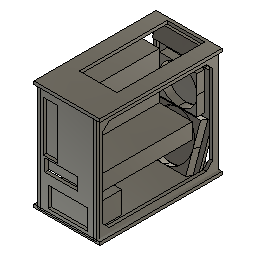
case (Autodesk Fusion 360 design; units mm, degrees)
Autodesk Fusion 360 part; units mm, degrees
sketch "Skizze1" plane through (0, 0, 0) normal (0, 1, 0) x (1, 0, 0)
  line L0 (-1.5, -33) -> (-1.5, -13)
  line L1 (-1.5, -13) -> (15.5, -13)
  line L2 (15.5, -13) -> (15.5, -18)
  line L3 (15.5, -18) -> (5, -18)
  line L4 (5, -18) -> (5, -33)
  line L5 (5, -33) -> (-1.5, -33)
  dimension "d1" = 20
  dimension "d2" = 17
  dimension "d3" = 5
  dimension "d4" = 10.5
  constraint vertical L0
  constraint perpendicular L0 L1
  constraint perpendicular L1 L2
  constraint perpendicular L0 L3
  constraint perpendicular L3 L4
  constraint perpendicular L0 L5
  measures "d1" distance of L0.start L0.end
  measures "d2" distance of L0.end L1.end
  measures "d3" distance of L1.end L2.end
  measures "d4" distance of L2.end L3.end
sketch "Skizze3" plane through (0, 0, 0) normal (1, 0, 0) x (0, 1, 0)
  line L0 (25, 35, -2) -> (-14, 35, -2)
  line L1 (-14, 35, -2) -> (-14, 1.5, -2)
  line L2 (-14, 1.5, -2) -> (25, 1.5, -2)
  line L3 (25, 1.5, -2) -> (25, 35, -2)
  line L4 (23, 31, -2) -> (21, 33, -2)
  line L5 (21, 33, -2) -> (-10, 33, -2)
  line L6 (-10, 33, -2) -> (-12, 31, -2)
  line L7 (-12, 31, -2) -> (-12, 5.5, -2)
  line L8 (-12, 5.5, -2) -> (-10, 3.5, -2)
  line L9 (-10, 3.5, -2) -> (21, 3.5, -2)
  line L10 (21, 3.5, -2) -> (23, 5.5, -2)
  line L11 (23, 5.5, -2) -> (23, 31, -2)
  line L12 (21, 33, -2) -> (23, 33, -2) construction
  line L13 (23, 31, -2) -> (23, 33, -2) construction
  line L14 (-12, 31, -2) -> (-12, 33, -2) construction
  line L15 (-12, 33, -2) -> (-10, 33, -2) construction
  line L16 (-12, 5.5, -2) -> (-12, 3.5, -2) construction
  line L17 (-12, 3.5, -2) -> (-10, 3.5, -2) construction
  line L18 (21, 3.5, -2) -> (23, 3.5, -2) construction
  line L19 (23, 3.5, -2) -> (23, 5.5, -2) construction
  dimension "d32" = 39
  dimension "height" = 33.5
  dimension "d34" = 29.5
  dimension "d35" = 35
  dimension "d36" = 2
  dimension "d37" = 2
  dimension "d38" = 2
  dimension "d39" = 2
  dimension "d40" = 2
  dimension "d41" = 2
  dimension "d42" = 2
  dimension "d43" = 2
sketch "Skizze4" plane through (0, 0, 0) normal (0, 0, 1) x (1, 0, 0)
  line L0 (-3, 25, 2) -> (18, 25, 2)
  line L1 (18, 25, 2) -> (18, -14, 2)
  line L2 (18, -14, 2) -> (-3, -14, 2)
  line L3 (-3, -14, 2) -> (-3, 25, 2)
  line L4 (13.5, -4, 2) -> (1.5, -4, 2)
  line L5 (1.5, -4, 2) -> (1.5, 24, 2)
  line L6 (1.5, 24, 2) -> (13.5, 24, 2)
  line L7 (13.5, 24, 2) -> (13.5, -4, 2)
  dimension "length" = 39
  dimension "width" = 21
sketch "Skizze5" plane through (0, 0, 0) normal (0, 1, 0) x (1, 0, 0)
  line L0 (-2, -35, -5) -> (17, -35, -5)
  line L1 (17, -35, -5) -> (17, -1.5, -5)
  line L2 (17, -1.5, -5) -> (-2, -1.5, -5)
  line L3 (-2, -1.5, -5) -> (-2, -35, -5)
  line L4 (14, -3, -5) -> (1.5, -3, -5)
  line L5 (1.5, -3, -5) -> (1.5, -9.5, -5)
  line L6 (1.5, -9.5, -5) -> (14, -9.5, -5)
  line L7 (14, -9.5, -5) -> (14, -3, -5)
  line L8 (0, -33, -5) -> (4.5, -33, -5)
  line L9 (4.5, -33, -5) -> (4.5, -17, -5)
  line L10 (4.5, -17, -5) -> (0, -17, -5)
  line L11 (0, -17, -5) -> (0, -33, -5)
  line L12 (0.5, -16.5, -5) -> (11, -16.5, -5)
  line L13 (11, -16.5, -5) -> (11, -12.5, -5)
  line L14 (11, -12.5, -5) -> (0.5, -12.5, -5)
  line L15 (0.5, -12.5, -5) -> (0.5, -16.5, -5)
  line L16 (14, -2, -5) -> (1, -2, -5)
  line L17 (1, -2, -5) -> (1, -9, -5)
  line L18 (1, -9, -5) -> (14, -9, -5)
  line L19 (14, -9, -5) -> (14, -2, -5)
  line L20 (18, -2) -> (-3, -2)
  dimension "d9" = 12.5
  dimension "d10" = 6.5
  dimension "d11" = 16
  dimension "d12" = 4.5
  dimension "d13" = 10.5
  dimension "d14" = 4
  dimension "d70" = 21
  dimension "d71" = 33.5
  measures "d70" distance of L20.start L20.end
sketch "Skizze6" plane through (0, 0, 0) normal (1, 0, 0) x (0, 1, 0)
  line L0 (25, 15.1374, -1) -> (20.2117, 1.9817, -1)
  line L1 (24, 15.1374, -1) -> (19.2117, 1.9817, -1)
  line L2 (24, 15.1374, -1) -> (24, 29.1374, -1)
  line L3 (19.2117, 1.9817, -1) -> (20.2117, 1.9817, -1)
  line L4 (25, 29.1374, -1) -> (25, 15.1374, -1)
  line L5 (22.851, 31.0958, -1) -> (24.3572, 35.234, -1)
  line L6 (24.2721, 35, -1) -> (23.1436, 35, -1)
  line L7 (23.1436, 35, -1) -> (21.7147, 31.074, -1)
  line L8 (24, 29.1323, -1) -> (21.7147, 31.074, -1)
  line L9 (25, 29.1374, -1) -> (22.851, 31.0958, -1)
  dimension "fansize" = 14
  dimension "d19" = 14
  dimension "d62" = 14
  dimension "d63" = 14
extrude "Extrusion2" add sketch "Skizze1" along normal blind 31 makes body 1
move_body "Verschieben3" bodies 1 to x (1, 0, 0) y (0, 1, 0) z (0, 0, 1) at (0, -4, 0)
extrude "Extrusion6" add sketch "Skizze5" along normal blind 1 separate body contours L0 L1 L2 L3 | L4 L5 L16 L17 L18 L19 in plane through (0, -5, 0) normal (0, 1, 0) makes body 2
move_body "Verschieben4" bodies 2 1 to x (1, 0, 0) y (0, 1, 0) z (0, 0, 1) at (0, -9, 0)
extrude "Extrusion3" add sketch "Skizze4" along normal blind 1 separate body contours L0 L1 L2 L3 in plane through (0, 0, 2) normal (0, 0, 1) makes body 3
move_body "Verschieben1" bodies 3 to x (1, 0, 0) y (0, 1, 0) z (0, 0, 1) at (0, 0, 33)
extrude "Extrusion4" add sketch "Skizze4" against normal blind 1 separate body contours L0 L1 L2 L3 | L4 L5 L6 L7 in plane through (0, 0, 2) normal (0, 0, 1) makes body 4
extrude "Extrusion5" add sketch "Skizze3" along normal blind 1 separate body contours L0 L1 L2 L3 in plane through (-2, 0, 0) normal (1, 0, 0) makes body 5
copy_body "Körper kopieren/einfügen1" bodies 5 makes body 6
move_body "Verschieben2" bodies 6 to x (1, 0, 0) y (0, 1, 0) z (0, 0, 1) at (18, 0, 0)
extrude "Extrusion7" add sketch "Skizze6" along normal blind 17 separate body contours L0 L1 L2 L3 L4 L5 L6 L7 L8 L9 in plane through (-1, 0, 0) normal (1, 0, 0) makes body 7
sketch "Skizze8" plane through (0, 16.3275, -5.9427) normal (0, -0.939693, 0.34202) x (1, 0, 0)
  line L0 (-1, 22.433) -> (-1, 8.433)
  line L1 (-1, 8.433) -> (16, 8.433)
  line L2 (16, 8.433) -> (16, 22.433)
  line L3 (16, 22.433) -> (-1, 22.433)
  circle A0 centre (7.5, 15.5) radius 7
  line L4 (0.5, 22.5) -> (14.5, 22.5)
  line L5 (14.5, 22.5) -> (14.5, 8.5)
  line L6 (14.5, 8.5) -> (0.5, 8.5)
  line L7 (0.5, 8.5) -> (0.5, 22.5)
  dimension "d57" = 14
  constraint horizontal L4
  constraint vertical L5
  constraint horizontal L6
  constraint vertical L7
  measures "d57" diameter of A0
extrude "Extrusion11" add sketch "Skizze8" along normal blind 2.5 separate body contours L3 A0 L4 L7 | L3 A0 L7 | A0 L6 L7 | L3 A0 L4 L5 | L3 A0 L5 | A0 L5 L6 makes body 8
extrude "Extrusion12" add sketch "Skizze5" along normal blind 10 separate body contours L4 L5 L7 L18 L19 | L4 L5 L16 L17 L18 L19 in plane through (0, -5, 0) normal (0, 1, 0) makes body 9
move_body "Verschieben5" bodies 9 to x (1, 0, 0) y (0, 1, 0) z (0, 0, 1) at (0, -8, 0)
sketch "Skizze9" plane through (0, 24, 0) normal (0, -1, 0) x (1, 0, 0)
  line L0 (-1, 29.1323) -> (-1, 15.1374)
  line L1 (-1, 15.1374) -> (16, 15.1374)
  line L2 (16, 15.1374) -> (16, 29.1323)
  line L3 (1.5, 28.5) -> (13.5, 28.5)
  line L4 (13.5, 28.5) -> (13.5, 16.5)
  line L5 (13.5, 16.5) -> (1.5, 16.5)
  line L6 (1.5, 16.5) -> (1.5, 28.5)
  circle A0 centre (7.5, 22.5) radius 6
  line L7 (16, 29.1323) -> (-1, 29.1323)
  dimension "d65" = 12
  dimension "d66" = 12
  dimension "d67" = 12
  constraint horizontal L3
  constraint vertical L4
  constraint horizontal L5
  constraint vertical L6
  measures "d65" distance of L3.start L3.end
  measures "d66" distance of L3.start L5.end
  measures "d67" diameter of A0
extrude "Extrusion13" add sketch "Skizze9" along normal blind 2.5 separate body contours L3 L6 A0 | L3 L4 A0 | L5 L6 A0 | L4 L5 A0 makes body 10
equation "d19 = fansize"
equation "d22 = thickness"
equation "d24 = -thickness"
equation "d26 = thickness"
equation "thickness = 1 mm"
equation "d32 = length"
equation "d34 = height - 4 mm"
equation "d35 = length - 4 mm"
equation "d44 = width - 4 mm"
equation "fan_thickness = 2.50 mm"
equation "d71 = height"
named bodies: "board", "top", "bottom", "side1", "side2", "back", "front", "fan", "powersupply", "fanhigh"
